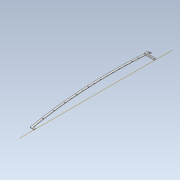
# Autodesk Inventor part: os_traverse
Saved by Autodesk Inventor 2020 (Build 240168000, 168)
## iProperties
Created: 2020-09-10
Part Number: os_traverse
Material: Generic
Document SubType Name: Modeling
Designer: Admin
Density: 1 g/cm^3
Appearance: Default
Author: Admin
Autodesk Inventor part; units mm, degrees
ref_plane "YZ Plane" through (0, 0, 0) normal (1, 0, 0) x (0, 1, 0)
ref_plane "XZ Plane" through (0, 0, 0) normal (0, 1, 0) x (-1, 0, 0)
ref_plane "XY Plane" through (0, 0, 0) normal (0, 0, 1) x (1, 0, 0)
sketch "Sketch1" plane through (0, 0, 0) normal (0, 1, 0) x (-1, 0, 0)
  line L0 (0, 0) -> (25, 0)
  line L1 (0, 0) -> (0, -10)
  line L2 (0, -10) -> (15, -10)
  line L3 (55, -790) -> (0, -790)
  line L4 (0, -790) -> (0, -800)
  line L5 (0, -800) -> (65, -800)
  arc A0 (65, -800) -> (25, 0) centre (-3125.8775, -558.5439) ccw
  arc A1 (55, -790) -> (15, -10) centre (-3125.8948, -562.0972) ccw
  line L6 (0, -960.2513) -> (0, 161.5078) projected
  dimension "d0" = 10
  dimension "d1" = 25
  dimension "d2" = 15
  dimension "d3" = 10
  dimension "d4" = 65
  dimension "d5" = 55
  dimension "d6" = 0
  dimension "d7" = 800
  dimension "d8" = 3200
  dimension "d9" = 3189.0486
  constraints: 12 end point, 4 point on circle, 3 perpendicular, 2 centre point, 2 horizontal, 1 vertical
  measures "d0" distance of L0.start L1.end
  measures "d1" distance of L0.start L0.end
  measures "d2" distance of L1.end L2.end
  measures "d3" distance of L3.end L4.end
  measures "d4" distance of L4.end L5.end
  measures "d5" distance of L3.start L3.end
  measures "d6" distance from line of L4 L1.end
  measures "d7" distance between parallel lines of L5 L0
  measures "d8" radius of A0
  measures "d9" radius of A1
extrude "Extrusion2" add sketch "Sketch1" along normal blind 3 contours L0 A0 L5 L4 L3 A1 L2 L1
sketch "Sketch3" plane through (0, 0, 0) normal (0, -1, 0) x (1, 0, 0)
  line L0 (-55, -790) -> (0, -790) projected
  line L1 (0, -790) -> (-63.7434, -790)
  line L2 (-63.7434, -790) -> (-63.7434, -770)
  line L3 (-63.7434, -770) -> (0, -770)
  line L4 (0, -770) -> (0, -790)
  point P0 (0, 0)
  dimension "d15" = 20
  dimension "d16" = 63.7434
  constraints: 8 end point, 2 parallel, 1 horizontal, 1 perpendicular
  measures "d15" distance of L1.end L2.end
  measures "d16" distance of L0.end L1.end
extrude "Extrusion3" add sketch "Sketch3" against normal blind 10
sketch "Sketch4" plane through (0, 0, 0) normal (0, -1, 0) x (1, 0, 0)
  arc A0 (-55, -776.2588) -> (0, -831.2588) centre (0, -776.2588) ccw
  line L0 (0, -831.2588) -> (0, -776.2588)
  line L1 (0, -776.2588) -> (-55, -776.2588)
  line L2 (0, -800) -> (0, -770) projected
  point P0 (0, 0)
  dimension "d19" = 0
  dimension "d20" = 0
  dimension "d21" = 55
  constraints: 4 end point, 2 point on circle, 1 centre point, 1 point on line
  measures "d19" horizontal distance of L0.end L0.start
  measures "d20" vertical distance of L1.end L0.end
  measures "d21" radius of A0
extrude "Extrusion4" cut sketch "Sketch4" against normal blind 10
fillet "Fillet1" radius 16 1 edges at (-65, 1.5, -800)
sketch "Sketch5" plane through (0, 0, 0) normal (0, -1, 0) x (1, 0, 0)
  line L0 (-65, -730) -> (0, -730)
  line L1 (0, -730) -> (0, -727)
  line L2 (0, -727) -> (-65, -727)
  line L3 (-65, -727) -> (-65, -730)
  line L4 (0, -770) -> (-56.3698, -770) projected
  line L5 (0, -776.2588) -> (0, -770) projected
  point P0 (0, 0)
  dimension "d25" = 3
  dimension "d26" = 40
  dimension "d27" = 65
  dimension "d28" = 0
  constraints: 8 end point, 2 parallel, 1 horizontal, 1 perpendicular
  measures "d25" distance of L0.end L1.end
  measures "d26" distance between parallel lines of L4 L0
  measures "d27" distance between parallel lines of L3 L5
  measures "d28" distance between parallel lines of L1 L5
extrude "Extrusion5" cut sketch "Sketch5" against normal blind 10
pattern_linear "Rectangular Pattern1" count 9 spacing 40 along (0, 0, 1) of "Extrusion5"
sketch "Sketch6" plane through (0, 0, 0) normal (0, -1, 0) x (1, 0, 0)
  line L0 (0, -370) -> (-60, -370)
  line L1 (-60, -370) -> (-60, -367)
  line L2 (-60, -367) -> (0, -367)
  line L3 (0, -367) -> (0, -370)
  line L4 (0, 0) -> (0, -10) projected
  line L5 (-59.5248, -410) -> (-65, -410) projected
  dimension "d34" = 3
  dimension "d35" = 0
  dimension "d36" = 40
  dimension "d37" = 60
  constraints: 8 end point, 2 parallel, 1 horizontal, 1 perpendicular
  measures "d34" distance of L0.end L1.end
  measures "d35" distance between parallel lines of L4 L3
  measures "d36" distance between parallel lines of L0 L5
  measures "d37" distance of L0.start L0.end
extrude "Extrusion6" cut sketch "Sketch6" against normal blind 10
pattern_linear "Rectangular Pattern2" count 2 spacing 40 along (0, 0, 1) of "Extrusion6"
sketch "Sketch7" plane through (0, 0, 0) normal (0, -1, 0) x (1, 0, 0)
  line L0 (0, -290) -> (-53, -290)
  line L1 (-53, -290) -> (-53, -287)
  line L2 (-53, -287) -> (0, -287)
  line L3 (0, -287) -> (0, -290)
  line L4 (0, -960) -> (0, 160) projected
  line L5 (-54.6967, -330) -> (-60, -330) projected
  point P0 (0, 0)
  dimension "d43" = 3
  dimension "d44" = 0
  dimension "d45" = 40
  dimension "d46" = 53
  constraints: 8 end point, 2 parallel, 1 horizontal, 1 perpendicular
  measures "d43" distance of L0.end L1.end
  measures "d44" distance from line of L0.start L4
  measures "d45" distance between parallel lines of L5 L0
  measures "d46" distance of L0.start L0.end
extrude "Extrusion7" cut sketch "Sketch7" against normal blind 10
pattern_linear "Rectangular Pattern3" count 2 spacing 40 along (0, 0, 1) of "Extrusion7"
sketch "Sketch8" plane through (0, 0, 0) normal (0, -1, 0) x (1, 0, 0)
  line L0 (0, -210) -> (-45, -210)
  line L1 (-45, -210) -> (-45, -207)
  line L2 (-45, -207) -> (0, -207)
  line L3 (0, -207) -> (0, -210)
  line L4 (-47.8454, -250) -> (-53, -250) projected
  line L5 (0, 0) -> (0, -10) projected
  dimension "d52" = 3
  dimension "d53" = 40
  dimension "d54" = 0
  dimension "d55" = 45
  constraints: 8 end point, 2 parallel, 1 horizontal, 1 perpendicular
  measures "d52" distance of L0.end L1.end
  measures "d53" distance between parallel lines of L4 L0
  measures "d54" distance between parallel lines of L5 L3
  measures "d55" distance of L0.start L0.end
extrude "Extrusion8" cut sketch "Sketch8" against normal blind 10
pattern_linear "Rectangular Pattern4" count 2 spacing 40 along (0, 0, 1) of "Extrusion8"
sketch "Sketch9" plane through (0, 0, 0) normal (0, -1, 0) x (1, 0, 0)
  line L0 (0, -90) -> (-35, -90)
  line L1 (-35, -90) -> (-35, -87)
  line L2 (-35, -87) -> (0, -87)
  line L3 (0, -87) -> (0, -90)
  line L4 (0, -10) -> (-15, -10) projected
  line L5 (0, 0) -> (0, -10) projected
  dimension "d61" = 3
  dimension "d62" = 77
  dimension "d63" = 0
  dimension "d64" = 35
  constraints: 8 end point, 2 parallel, 1 horizontal, 1 perpendicular
  measures "d61" distance of L0.end L1.end
  measures "d62" distance between parallel lines of L4 L2
  measures "d63" distance between parallel lines of L5 L3
  measures "d64" distance of L0.start L0.end
extrude "Extrusion9" cut sketch "Sketch9" against normal blind 10
body "Solid2"
